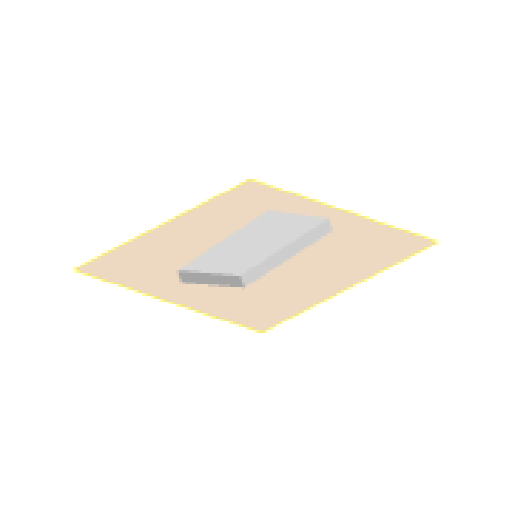
# Autodesk Inventor part: Грунт
Saved by Autodesk Inventor 2026 (Build 300175000, 175)
## iProperties
Created: 2026-05-26
Part Number: Грунт
Material: Типовые
Document SubType Name: Modeling
Designer: Artem Sannikov
Density: 1 g/cm^3
Appearance: По умолчанию
Author: Artem Sannikov
Autodesk Inventor part; units mm, degrees
ref_plane "YZ Plane" through (0, 0, 0) normal (1, 0, 0) x (0, 1, 0)
ref_plane "XZ Plane" through (0, 0, 0) normal (0, 1, 0) x (-1, 0, 0)
ref_plane "XY Plane" through (0, 0, 0) normal (0, 0, 1) x (1, 0, 0)
ref_plane "РабПлоскость1" through (242.0717, -244.4536, 149.7988) normal (-0.3714, 0.9276, 0.0392) x (-0.9113, -0.3562, -0.2065)
sketch "Эскиз1" plane through (242.0717, -244.4536, 149.7988) normal (-0.3714, 0.9276, 0.0392) x (-0.9113, -0.3562, -0.2065)
  line L0 (38.9879, 72.7933) -> (-26.7023, 56.0578)
  line L1 (63.689, -24.1634) -> (38.9879, 72.7933)
  line L2 (-26.7023, 56.0578) -> (-5.4683, -37.5395)
  line L3 (-5.4683, -37.5395) -> (63.689, -24.1634)
  point P0 (164.4728, -130.9329)
  constraints: 8 end point, 8 other
extrude "Выдавливание1" add sketch "Эскиз1" along normal blind 10
